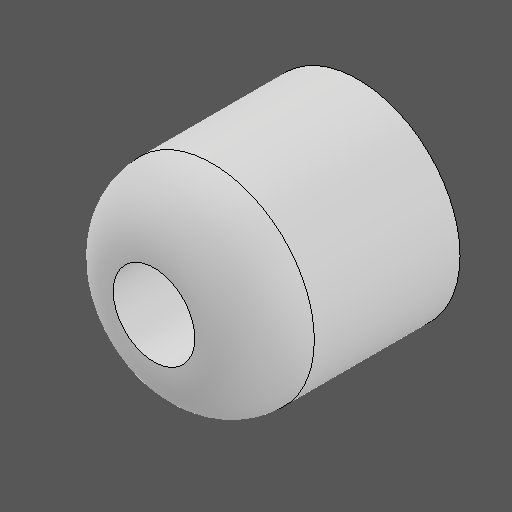
# Autodesk Inventor part: Ceramic-scaler-7x2.8x7
Saved by Autodesk Inventor 2025 (Build 290162000, 162)
## iProperties
Created: 2024-05-30
Part Number: Ceramic-scaler-7x2.8x7
Material: Generic
Document SubType Name: Modeling
Designer: kuzmin
Density: 1 g/cm^3
Appearance: Default
Author: kuzmin
Autodesk Inventor part; units mm, degrees
ref_plane "YZ Plane" through (0, 0, 0) normal (1, 0, 0) x (0, 1, 0)
ref_plane "XZ Plane" through (0, 0, 0) normal (0, 1, 0) x (-1, 0, 0)
ref_plane "XY Plane" through (0, 0, 0) normal (0, 0, 1) x (1, 0, 0)
sketch "Sketch1" plane through (0, 0, 0) normal (0, 1, 0) x (-1, 0, 0)
  line L0 (3.5, 0) -> (3.5, 5)
  line L1 (1.4, 1.5) -> (1.4, 7)
  arc A0 (3.5, 5) -> (1.4, 7) centre (1.4976, 5) ccw
  arc A1 (3.5, 0) -> (1.4, 1.5) centre (1.5618, -0.4934) ccw
  line L2 (0, 0) -> (0, 8.4077)
  dimension "d0" = 2.8
  dimension "d1" = 7
  dimension "d2" = 7
  dimension "d3" = 5
  dimension "d4" = 5.5
  dimension "d5" = 2
  constraints: 6 end point, 4 point on circle, 3 vertical, 2 centre point, 1 horizontal alignment, 1 tangent
  measures "d0" diameter of L1 L2
  measures "d1" diameter of L0 L2
  measures "d2" vertical distance of L1.end L0.start
  measures "d3" distance of L0.start L0.end
  measures "d4" distance of L1.start L1.end
  measures "d5" radius of A1
revolve "Revolution1" add sketch "Sketch1" angle 360 about axis through (0, 0, 0) along (0, 0, 1)
body "Solid1"
